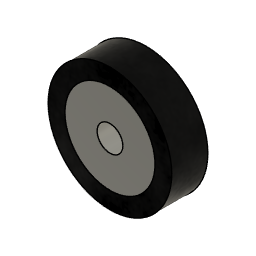
Wheel 2 v1 (Autodesk Fusion 360 design; units mm, degrees)
Autodesk Fusion 360 part; units mm, degrees
sketch "Sketch1" plane through (0, 0, 0) normal (0, 1, 0) x (1, 0, 0)
  circle A0 centre (0, 0) radius 8.75
  dimension "d1" = 17.5
  constraint coincident A0.centre origin
  measures "d1" diameter of A0
extrude "Extrude1" add sketch "Sketch1" along normal blind 7 makes body 1
sketch "Sketch2" plane through (0, 0, 0) normal (0, 1, 0) x (1, 0, 0)
  circle A0 centre (0, 0) radius 12
  circle A1 centre (0, 0) radius 8.75
  dimension "d4" = 24
  dimension "d5" = 17.5
  constraint coincident A0.centre A1.centre
  measures "d4" diameter of A0
  measures "d5" diameter of A1
extrude "Extrude2" add sketch "Sketch2" along normal blind 7 separate body makes body 2
sketch "Sketch3" plane through (0, 0, 0) normal (0, -1, 0) x (1, 0, 0)
  circle A0 centre (0, 0) radius 8.75
  circle A1 centre (0, 0) radius 2.5
  dimension "d8" = 5
  constraint concentric A0 A1
  measures "d8" diameter of A1
extrude "Extrude3" cut sketch "Sketch3" against normal blind 39 contours A1 bodies 1
